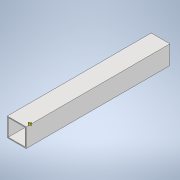
# Autodesk Inventor part: 4_barra
Saved by Autodesk Inventor 2020 (Build 240168000, 168)
## iProperties
Created: 2019-10-11
Part Number: 4_barra
Material: Generico
Document SubType Name: Modeling
Designer: socci
Density: 1 g/cm^3
Appearance: Default
Author: socci
Autodesk Inventor part; units mm, degrees
ref_plane "YZ Plane" through (0, 0, 0) normal (1, 0, 0) x (0, 1, 0)
ref_plane "XZ Plane" through (0, 0, 0) normal (0, 1, 0) x (-1, 0, 0)
ref_plane "XY Plane" through (0, 0, 0) normal (0, 0, 1) x (1, 0, 0)
sketch "Schizzo1" plane through (0, 0, 0) normal (0, 0, 1) x (1, 0, 0)
  line L0 (10, -10) -> (-10, -10)
  line L1 (-10, -10) -> (-10, 10)
  line L2 (-10, 10) -> (10, 10)
  line L3 (10, 10) -> (10, -10)
  line L4 (9, 9) -> (-9, 9)
  line L5 (-9, 9) -> (-9, -9)
  line L6 (-9, -9) -> (9, -9)
  line L7 (9, -9) -> (9, 9)
  point P0 (0, 0)
  point P1 (0, 0)
  dimension "d0" = 20
  dimension "d1" = 1
  constraints: 16 end point, 1 coincident, 12 other
  measures "d0" distance of L1.end L2.end
  measures "d1" distance between parallel lines of L2 L4
extrude "Estrusione1" add sketch "Schizzo1" against normal blind 153
